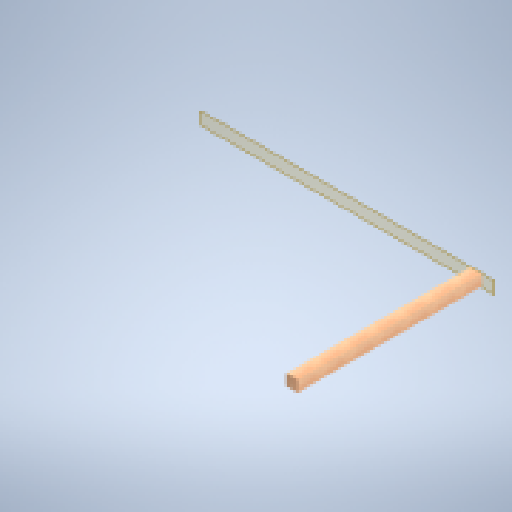
# Autodesk Inventor part: 4x4x66
Saved by Autodesk Inventor 2025 (Build 290162000, 162)
## iProperties
Created: 2024-09-03
Part Number: 4x4x66
Material: Wood (Birch)
Document SubType Name: Modeling
Designer: Win
Density: 0.55 g/cm^3
Appearance: Birch - Natural Polished
Author: Win
Autodesk Inventor part; units mm, degrees
ref_plane "YZ Plane" through (0, 0, 0) normal (1, 0, 0) x (0, 1, 0)
ref_plane "XZ Plane" through (0, 0, 0) normal (0, 1, 0) x (-1, 0, 0)
ref_plane "XY Plane" through (0, 0, 0) normal (0, 0, 1) x (1, 0, 0)
ref_plane "Work Plane2" through (8054.1679, 131.4642, -2407.6713) normal (0, 0, 1) x (0, 1, 0)
sketch "Sketch1" plane through (8054.1679, 131.4642, -2407.6713) normal (0, 0, 1) x (0, 1, 0)
  line L0 (0, -0.8466) -> (101.6, -0.8466)
  line L1 (101.6, -0.8466) -> (101.6, 100.7534)
  line L2 (101.6, 100.7534) -> (0, 100.7534)
  line L3 (0, 100.7534) -> (0, -0.8466)
  point P0 (-131.4642, 8054.1679)
  dimension "d0" = 101.6
  dimension "d1" = 101.6
  constraints: 8 end point, 2 parallel, 1 horizontal, 1 perpendicular
  measures "d0" distance of L2.end L1.end
  measures "d1" distance of L0.end L1.end
extrude "Extrusion1" add sketch "Sketch1" along normal blind 1676.4
body "Solid1"
